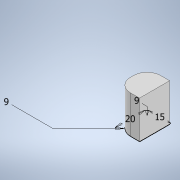
# Autodesk Inventor part: actuator_tube_test
Saved by Autodesk Inventor 2021 (Build 250183000, 183)
## iProperties
Created: 2021-04-28
Part Number: actuator_tube_test
Material: Generic
Document SubType Name: Modeling
Designer: Charlie
Density: 1 g/cm^3
Appearance: Default
Author: Charlie
Autodesk Inventor part; units mm, degrees
ref_plane "YZ Plane" through (0, 0, 0) normal (1, 0, 0) x (0, 1, 0)
ref_plane "XZ Plane" through (0, 0, 0) normal (0, 1, 0) x (-1, 0, 0)
ref_plane "XY Plane" through (0, 0, 0) normal (0, 0, 1) x (1, 0, 0)
sketch "Sketch1" plane through (0, 0, 0) normal (0, 1, 0) x (-1, 0, 0)
  line L0 (-7.5, 10) -> (-1.5, 10)
  line L1 (7.5, 1) -> (7.5, -1)
  line L2 (-1.5, -10) -> (-7.5, -10)
  line L3 (-7.5, -10) -> (-7.5, 10)
  line L4 (-7.5, 10) -> (7.5, -10) construction
  line L5 (7.5, 10) -> (-7.5, -10) construction
  arc A0 (7.5, 1) -> (-1.5, 10) centre (-1.5, 1) ccw
  arc A1 (-1.5, -10) -> (7.5, -1) centre (-1.5, -1) ccw
  point P0 (0, 0)
  dimension "d0" = 15
  dimension "d1" = 20
  dimension "d4" = 9
  dimension "d5" = 9
  constraints: 12 end point, 4 point on circle, 4 point on line, 4 tangent, 2 centre point, 2 midpoint, 2 parallel, 1 horizontal, 1 perpendicular
  measures "d0" distance of L4.end L2.end
  measures "d1" distance of L5.start L4.end
  measures "d4" radius of A0
  measures "d5" radius of A1
extrude "Extrusion1" add sketch "Sketch1" along normal blind 25
shell "Shell1" thickness 1 removed faces 1 at (-1.5, 0, 0.3333)
extrude "Extrusion2" add sketch "Sketch1" along normal blind 1
body "Solid1"
